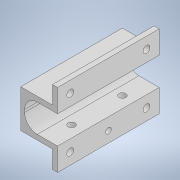
# Autodesk Inventor part: Part3
Saved by Autodesk Inventor 2022 (Build 260153000, 153)
## iProperties
Created: 2022-12-27
Part Number: Part3
Material: Generic
Document SubType Name: Modeling
Designer: Gaming
Density: 1 g/cm^3
Appearance: Default
Author: Gaming
Autodesk Inventor part; units mm, degrees
ref_plane "YZ Plane" through (0, 0, 0) normal (1, 0, 0) x (0, 1, 0)
ref_plane "XZ Plane" through (0, 0, 0) normal (0, 1, 0) x (-1, 0, 0)
ref_plane "XY Plane" through (0, 0, 0) normal (0, 0, 1) x (1, 0, 0)
sketch "Sketch1" plane through (0, 0, 0) normal (0, 0, 1) x (1, 0, 0)
  line L0 (0, 0) -> (-29, 0)
  line L1 (-29, 0) -> (-29, 4)
  line L2 (-29, 4) -> (-4, 4)
  line L3 (-4, 4) -> (-4, 18)
  line L4 (-4, 18) -> (0, 18)
  line L5 (0, 18) -> (0, 0)
  dimension "d0" = 4
  dimension "d1" = 4
  dimension "d2" = 29
  dimension "d3" = 18
  constraints: 12 end point, 5 perpendicular, 1 horizontal
  measures "d0" distance of L3.end L4.end
  measures "d1" distance between parallel lines of L0 L2
  measures "d2" distance between parallel lines of L1 L5
  measures "d3" distance between parallel lines of L0 L4
extrude "Extrusion1" add sketch "Sketch1" along normal blind 80
sketch "Sketch3" plane through (0, 0, 0) normal (1, 0, 0) x (0, 0, -1)
  line L0 (0, 0) -> (-80, 0) projected
  line L1 (-80, 0) -> (-80, 18) projected
  line L2 (0, 0) -> (0, 18) projected
  point P0 (-70, 9)
  point P1 (-10, 9)
  dimension "d9" = 9
  dimension "d10" = 10
  dimension "d11" = 10
  constraints: 1 horizontal alignment
  measures "d9" distance from line of point (-70, 9) L0
  measures "d10" distance from line of point (-70, 9) L1
  measures "d11" distance from line of point (-10, 9) L2
hole "Hole1" at (0, 9, 70) at (0, 9, 10) direction (-1, 0, 0) diameter 5.5 end through all
sketch "Sketch4" plane through (-29, 0, 0) normal (0, -1, 0) x (1, 0, 0)
  line L0 (29, 0) -> (29, 80) projected
  line L1 (0, 0) -> (29, 0) projected
  point P0 (20, 60)
  point P1 (20, 20)
  dimension "d19" = 9
  dimension "d20" = 20
  dimension "d21" = 20
  constraints: 1 vertical alignment
  measures "d19" distance from line of point (20, 60) L0
  measures "d20" vertical distance of point (20, 60) L0.end
  measures "d21" distance from line of point (20, 20) L1
hole "Hole2" at (-9, 0, 60) at (-9, 0, 20) direction (0, 1, 0) diameter 5.5 end through all
sketch "Sketch9" plane through (-29, 0, 0) normal (0, -1, 0) x (1, 0, 0)
  line L0 (25, 80) -> (0, 80) projected
  line L1 (25, 0) -> (0, 0) projected
  line L2 (0, 80) -> (3, 80)
  line L3 (3, 80) -> (3, 0)
  line L4 (3, 0) -> (0, 0)
  line L5 (0, 0) -> (0, 80)
  point P0 (29, 0)
  point P1 (3, 80)
  dimension "d57" = 3
  constraints: 8 end point, 2 parallel, 1 horizontal, 1 perpendicular, 1 point on line
  measures "d57" distance of L2.end L0.end
extrude "Extrusion5" add sketch "Sketch9" along normal blind 26
sketch "Sketch10" plane through (-26, 0, 80) normal (1, 0, 0) x (0, 0, -1)
  line L0 (80, -26) -> (0, -26) projected
  line L1 (80, 4) -> (80, -26) projected
  line L2 (0, -26) -> (80, -26)
  line L3 (80, -26) -> (80, -22)
  line L4 (80, -22) -> (0, -22)
  line L5 (0, -22) -> (0, -26)
  point P0 (80, 0)
  dimension "d60" = 4
  constraints: 8 end point, 2 parallel, 1 horizontal, 1 perpendicular, 1 point on line
  measures "d60" distance of L3.end L0.start
extrude "Extrusion6" add sketch "Sketch10" along normal blind 26
sketch "Sketch11" plane through (-29, -26, 0) normal (0, -1, 0) x (1, 0, 0)
  line L0 (29, 80) -> (25, 80) projected
  line L1 (25, 0) -> (0, 0) projected
  line L2 (29, 80) -> (25, 80)
  line L3 (25, 80) -> (25, 0)
  line L4 (25, 0) -> (29, 0)
  line L5 (29, 0) -> (29, 80)
  point P0 (29, 0)
  dimension "d63" = 4
  constraints: 8 end point, 2 parallel, 1 horizontal, 1 perpendicular, 1 point on line
  measures "d63" distance of L0.start L2.end
extrude "Extrusion7" add sketch "Sketch11" along normal blind 14
sketch "Sketch12" plane through (0, 0, 80) normal (1, 0, 0) x (0, 0, -1)
  circle A0 centre (10, 9) radius 2.75 projected
  circle A1 centre (70, 9) radius 2.75 projected
  line L0 (80, 18) -> (0, 18) projected
  line L1 (80, -40) -> (0, -40) projected
  line L2 (80, -22) -> (0, -22) projected
  point P0 (80, 0)
  point P1 (10, -31)
  point P2 (70, -31)
  point P3 (51, 18)
  dimension "d66" = 9
  dimension "d85" = 9
  constraints: 2 vertical alignment, 1 horizontal alignment
  measures "d66" distance from line of L0 A1.centre
  measures "d85" distance from line of L2 point (10, -31)
hole "Hole5" at (0, -31, 70) at (0, -31, 10) direction (-1, 0, 0) diameter 5.5 end through all
sketch "Sketch14" plane through (-26, -22, 80) normal (0, 1, 0) x (1, 0, 0)
  circle A0 centre (17, 20) radius 2.75 projected
  circle A1 centre (17, 60) radius 2.75 projected
  point P0 (26, 80)
  constraints: 2 coincident
hole "Hole6" at (-9, -22, 60) at (-9, -22, 20) direction (0, -1, 0) diameter 5.5 end through all
sketch "Sketch24" plane through (0, 0, 80) normal (1, 0, 0) x (0, 0, -1)
  line L0 (80, -40) -> (0, -40) projected
  line L1 (0, -22) -> (0, -40) projected
  point P0 (80, 0)
  point P1 (40, -31.5)
  dimension "d157" = 8.5
  dimension "d158" = 40
  measures "d157" distance from line of L0 point (40, -31.5)
  measures "d158" distance from line of L1 point (40, -31.5)
hole "Hole9" at (0, -31.5, 40) direction (-1, 0, 0) diameter 4.5 depth 8 tip angle 118
fillet "Fillet1" radius 10 2 edges at (-26, -22, 40) (-26, 0, 40)
equation "\"d11\" = d10"
equation "\"d21\" = d20"
body "Solid1"
